Autodesk Fusion 360 part; units mm, degrees
(part 4 of 5)
  line L264 (61.2673, -37.956) -> (48.2686, -37.956)
  spline S265 degree 3 poles (48.2686, -37.956) (47.9937, -37.956) (47.7687, -37.7311) (47.7687, -37.456) knots 6 6 6 6 7 7 7 7
  line L265 (47.7687, -37.456) -> (47.7687, -24.4562)
  spline S266 degree 3 poles (4.9055, 32.6938) (4.9055, 32.9689) (5.1304, 33.1939) (5.4054, 33.1939) knots 0 0 0 0 1 1 1 1
  line L266 (5.4054, 33.1939) -> (18.4054, 33.1939)
  spline S267 degree 3 poles (18.4054, 33.1939) (18.6807, 33.1939) (18.9057, 32.9689) (18.9057, 32.6938) knots 2 2 2 2 3 3 3 3
  line L267 (18.9057, 32.6938) -> (18.9057, 19.6941)
  spline S268 degree 3 poles (18.9057, 19.6941) (18.9057, 19.419) (18.6807, 19.194) (18.4054, 19.194) knots 4 4 4 4 5 5 5 5
  line L268 (18.4054, 19.194) -> (5.4054, 19.194)
  spline S269 degree 3 poles (5.4054, 19.194) (5.1304, 19.194) (4.9055, 19.419) (4.9055, 19.6941) knots 6 6 6 6 7 7 7 7
  line L269 (4.9055, 19.6941) -> (4.9055, 32.6938)
  line L270 (-4.6195, 0.6441) -> (-4.6195, 13.6438)
  spline S270 degree 3 poles (-4.6195, 13.6438) (-4.6195, 13.9189) (-4.3946, 14.1438) (-4.1196, 14.1438) knots 1 1 1 1 2 2 2 2
  line L271 (-4.1196, 14.1438) -> (8.8804, 14.1438)
  spline S271 degree 3 poles (8.8804, 14.1438) (9.1557, 14.1438) (9.3807, 13.9189) (9.3807, 13.6438) knots 3 3 3 3 4 4 4 4
  line L272 (9.3807, 13.6438) -> (9.3807, 0.6441)
  spline S272 degree 3 poles (9.3807, 0.6441) (9.3807, 0.369) (9.1557, 0.144) (8.8804, 0.144) knots 5 5 5 5 6 6 6 6
  line L273 (8.8804, 0.144) -> (-4.1196, 0.144)
  spline S273 degree 3 poles (-4.1196, 0.144) (-4.3946, 0.144) (-4.6195, 0.369) (-4.6195, 0.6441) knots 7 7 7 7 8 8 8 8
  spline S274 degree 3 poles (-14.1445, 56.506) (-14.1445, 56.7811) (-13.9196, 57.006) (-13.6447, 57.006) knots 0 0 0 0 1 1 1 1
  line L274 (-13.6447, 57.006) -> (-0.6446, 57.006)
  spline S275 degree 3 poles (-0.6446, 57.006) (-0.3693, 57.006) (-0.1443, 56.7811) (-0.1443, 56.506) knots 2 2 2 2 3 3 3 3
  line L275 (-0.1443, 56.506) -> (-0.1443, 43.5059)
  spline S276 degree 3 poles (-0.1443, 43.5059) (-0.1443, 43.2308) (-0.3693, 43.0058) (-0.6446, 43.0058) knots 4 4 4 4 5 5 5 5
  line L276 (-0.6446, 43.0058) -> (-13.6447, 43.0058)
  spline S277 degree 3 poles (-13.6447, 43.0058) (-13.9196, 43.0058) (-14.1445, 43.2308) (-14.1445, 43.5059) knots 6 6 6 6 7 7 7 7
  line L277 (-14.1445, 43.5059) -> (-14.1445, 56.506)
  spline S278 degree 3 poles (-52.2446, 56.506) (-52.2446, 56.7811) (-52.0196, 57.006) (-51.7447, 57.006) knots 0 0 0 0 1 1 1 1
  line L278 (-51.7447, 57.006) -> (-38.7446, 57.006)
  spline S279 degree 3 poles (-38.7446, 57.006) (-38.4693, 57.006) (-38.2444, 56.7811) (-38.2444, 56.506) knots 2 2 2 2 3 3 3 3
  line L279 (-38.2444, 56.506) -> (-38.2444, 43.5059)
  spline S280 degree 3 poles (-38.2444, 43.5059) (-38.2444, 43.2308) (-38.4693, 43.0058) (-38.7446, 43.0058) knots 4 4 4 4 5 5 5 5
  line L280 (-38.7446, 43.0058) -> (-51.7447, 43.0058)
  spline S281 degree 3 poles (-51.7447, 43.0058) (-52.0196, 43.0058) (-52.2446, 43.2308) (-52.2446, 43.5059) knots 6 6 6 6 7 7 7 7
  line L281 (-52.2446, 43.5059) -> (-52.2446, 56.506)
  line L282 (-71.5816, 13.6438) -> (-71.5816, 0.6441)
  spline S282 degree 3 poles (-71.5816, 0.6441) (-71.5816, 0.369) (-71.8065, 0.144) (-72.0818, 0.144) knots 1 1 1 1 2 2 2 2
  line L283 (-72.0818, 0.144) -> (-85.0819, 0.144)
  spline S283 degree 3 poles (-85.0819, 0.144) (-85.3568, 0.144) (-85.5817, 0.369) (-85.5817, 0.6441) knots 3 3 3 3 4 4 4 4
  line L284 (-85.5817, 0.6441) -> (-85.5817, 13.6438)
  spline S284 degree 3 poles (-85.5817, 13.6438) (-85.5817, 13.9189) (-85.3568, 14.1438) (-85.0819, 14.1438) knots 5 5 5 5 6 6 6 6
  line L285 (-85.0819, 14.1438) -> (-72.0818, 14.1438)
  spline S285 degree 3 poles (-72.0818, 14.1438) (-71.8065, 14.1438) (-71.5816, 13.9189) (-71.5816, 13.6438) knots 7 7 7 7 8 8 8 8
  spline S286 degree 3 poles (-57.0067, -5.4062) (-57.0067, -5.1311) (-56.7818, -4.9062) (-56.5068, -4.9062) knots 0 0 0 0 1 1 1 1
  line L286 (-56.5068, -4.9062) -> (-43.5068, -4.9062)
  spline S287 degree 3 poles (-43.5068, -4.9062) (-43.2315, -4.9062) (-43.0065, -5.1311) (-43.0065, -5.4062) knots 2 2 2 2 3 3 3 3
  line L287 (-43.0065, -5.4062) -> (-43.0065, -18.406)
  spline S288 degree 3 poles (-43.0065, -18.406) (-43.0065, -18.681) (-43.2315, -18.906) (-43.5068, -18.906) knots 4 4 4 4 5 5 5 5
  line L288 (-43.5068, -18.906) -> (-56.5068, -18.906)
  spline S289 degree 3 poles (-56.5068, -18.906) (-56.7818, -18.906) (-57.0067, -18.681) (-57.0067, -18.406) knots 6 6 6 6 7 7 7 7
  line L289 (-57.0067, -18.406) -> (-57.0067, -5.4062)
  spline S290 degree 3 poles (43.0055, 56.506) (43.0055, 56.7811) (43.2305, 57.006) (43.5054, 57.006) knots 0 0 0 0 1 1 1 1
  line L290 (43.5054, 57.006) -> (56.5055, 57.006)
  spline S291 degree 3 poles (56.5055, 57.006) (56.7807, 57.006) (57.0057, 56.7811) (57.0057, 56.506) knots 2 2 2 2 3 3 3 3
  line L291 (57.0057, 56.506) -> (57.0057, 43.5059)
  spline S292 degree 3 poles (57.0057, 43.5059) (57.0057, 43.2308) (56.7807, 43.0058) (56.5055, 43.0058) knots 4 4 4 4 5 5 5 5
  line L292 (56.5055, 43.0058) -> (43.5054, 43.0058)
  spline S293 degree 3 poles (43.5054, 43.0058) (43.2305, 43.0058) (43.0055, 43.2308) (43.0055, 43.5059) knots 6 6 6 6 7 7 7 7
  line L293 (43.0055, 43.5059) -> (43.0055, 56.506)
  spline S294 degree 3 poles (38.7436, -18.906) (38.4687, -18.906) (38.2437, -18.681) (38.2437, -18.406) knots 0 0 0 0 1 1 1 1
  line L294 (38.2437, -18.406) -> (38.2437, -5.4062)
  spline S295 degree 3 poles (38.2437, -5.4062) (38.2437, -5.1311) (38.4687, -4.9062) (38.7436, -4.9062) knots 2 2 2 2 3 3 3 3
  line L295 (38.7436, -4.9062) -> (51.7433, -4.9062)
  spline S296 degree 3 poles (51.7433, -4.9062) (52.0186, -4.9062) (52.2435, -5.1311) (52.2435, -5.4062) knots 4 4 4 4 5 5 5 5
  line L296 (52.2435, -5.4062) -> (52.2435, -18.406)
  spline S297 degree 3 poles (52.2435, -18.406) (52.2435, -18.681) (52.0186, -18.906) (51.7433, -18.906) knots 6 6 6 6 7 7 7 7
  line L297 (51.7433, -18.906) -> (38.7436, -18.906)
  spline S298 degree 3 poles (-33.1946, 56.506) (-33.1946, 56.7811) (-32.9696, 57.006) (-32.6947, 57.006) knots 0 0 0 0 1 1 1 1
  line L298 (-32.6947, 57.006) -> (-19.6946, 57.006)
  spline S299 degree 3 poles (-19.6946, 57.006) (-19.4193, 57.006) (-19.1944, 56.7811) (-19.1944, 56.506) knots 2 2 2 2 3 3 3 3
  line L299 (-19.1944, 56.506) -> (-19.1944, 43.5059)
  spline S300 degree 3 poles (-19.1944, 43.5059) (-19.1944, 43.2308) (-19.4193, 43.0058) (-19.6946, 43.0058) knots 4 4 4 4 5 5 5 5
  line L300 (-19.6946, 43.0058) -> (-32.6947, 43.0058)
  spline S301 degree 3 poles (-32.6947, 43.0058) (-32.9696, 43.0058) (-33.1946, 43.2308) (-33.1946, 43.5059) knots 6 6 6 6 7 7 7 7
  line L301 (-33.1946, 43.5059) -> (-33.1946, 56.506)
  spline S302 degree 3 poles (-176.3566, -37.456) (-176.3566, -37.7311) (-176.5816, -37.956) (-176.8568, -37.956) knots 0 0 0 0 1 1 1 1
  line L302 (-176.8568, -37.956) -> (-189.8569, -37.956)
  spline S303 degree 3 poles (-189.8569, -37.956) (-190.1318, -37.956) (-190.3568, -37.7311) (-190.3568, -37.456) knots 2 2 2 2 3 3 3 3
  line L303 (-190.3568, -37.456) -> (-190.3568, -24.4562)
  spline S304 degree 3 poles (-190.3568, -24.4562) (-190.3568, -24.1811) (-190.1318, -23.9562) (-189.8569, -23.9562) knots 4 4 4 4 5 5 5 5
  line L304 (-189.8569, -23.9562) -> (-176.8568, -23.9562)
  spline S305 degree 3 poles (-176.8568, -23.9562) (-176.5816, -23.9562) (-176.3566, -24.1811) (-176.3566, -24.4562) knots 6 6 6 6 7 7 7 7
  line L305 (-176.3566, -24.4562) -> (-176.3566, -37.456)
  spline S306 degree 3 poles (-176.3566, 0.6441) (-176.3566, 0.369) (-176.5816, 0.144) (-176.8568, 0.144) knots 0 0 0 0 1 1 1 1
  line L306 (-176.8568, 0.144) -> (-189.8569, 0.144)
  spline S307 degree 3 poles (-189.8569, 0.144) (-190.1318, 0.144) (-190.3568, 0.369) (-190.3568, 0.6441) knots 2 2 2 2 3 3 3 3
  line L307 (-190.3568, 0.6441) -> (-190.3568, 13.6438)
  spline S308 degree 3 poles (-190.3568, 13.6438) (-190.3568, 13.9189) (-190.1318, 14.1438) (-189.8569, 14.1438) knots 4 4 4 4 5 5 5 5
  line L308 (-189.8569, 14.1438) -> (-176.8568, 14.1438)
  spline S309 degree 3 poles (-176.8568, 14.1438) (-176.5816, 14.1438) (-176.3566, 13.9189) (-176.3566, 13.6438) knots 6 6 6 6 7 7 7 7
  line L309 (-176.3566, 13.6438) -> (-176.3566, 0.6441)
  spline S310 degree 3 poles (57.7936, -18.906) (57.5187, -18.906) (57.2937, -18.681) (57.2937, -18.406) knots 0 0 0 0 1 1 1 1
  line L310 (57.2937, -18.406) -> (57.2937, -5.4062)
  spline S311 degree 3 poles (57.2937, -5.4062) (57.2937, -5.1311) (57.5187, -4.9062) (57.7936, -4.9062) knots 2 2 2 2 3 3 3 3
  line L311 (57.7936, -4.9062) -> (70.7933, -4.9062)
  spline S312 degree 3 poles (70.7933, -4.9062) (71.0686, -4.9062) (71.2935, -5.1311) (71.2935, -5.4062) knots 4 4 4 4 5 5 5 5
  line L312 (71.2935, -5.4062) -> (71.2935, -18.406)
  spline S313 degree 3 poles (71.2935, -18.406) (71.2935, -18.681) (71.0686, -18.906) (70.7933, -18.906) knots 6 6 6 6 7 7 7 7
  line L313 (70.7933, -18.906) -> (57.7936, -18.906)
  spline S314 degree 3 poles (95.3937, -5.4062) (95.3937, -5.1311) (95.6187, -4.9062) (95.8936, -4.9062) knots 0 0 0 0 1 1 1 1
  line L314 (95.8936, -4.9062) -> (108.8933, -4.9062)
  spline S315 degree 3 poles (108.8933, -4.9062) (109.1686, -4.9062) (109.3936, -5.1311) (109.3936, -5.4062) knots 2 2 2 2 3 3 3 3
  line L315 (109.3936, -5.4062) -> (109.3936, -18.406)
  spline S316 degree 3 poles (109.3936, -18.406) (109.3936, -18.681) (109.1686, -18.906) (108.8933, -18.906) knots 4 4 4 4 5 5 5 5
  line L316 (108.8933, -18.906) -> (95.8936, -18.906)
  spline S317 degree 3 poles (95.8936, -18.906) (95.6187, -18.906) (95.3937, -18.681) (95.3937, -18.406) knots 6 6 6 6 7 7 7 7
  line L317 (95.3937, -18.406) -> (95.3937, -5.4062)
  line L318 (33.4805, 0.6441) -> (33.4805, 13.6438)
  spline S318 degree 3 poles (33.4805, 13.6438) (33.4805, 13.9189) (33.7055, 14.1438) (33.9804, 14.1438) knots 1 1 1 1 2 2 2 2
  line L319 (33.9804, 14.1438) -> (46.9805, 14.1438)
  spline S319 degree 3 poles (46.9805, 14.1438) (47.2557, 14.1438) (47.4807, 13.9189) (47.4807, 13.6438) knots 3 3 3 3 4 4 4 4
  line L320 (47.4807, 13.6438) -> (47.4807, 0.6441)
  spline S320 degree 3 poles (47.4807, 0.6441) (47.4807, 0.369) (47.2557, 0.144) (46.9805, 0.144) knots 5 5 5 5 6 6 6 6
  line L321 (46.9805, 0.144) -> (33.9804, 0.144)
  spline S321 degree 3 poles (33.9804, 0.144) (33.7055, 0.144) (33.4805, 0.369) (33.4805, 0.6441) knots 7 7 7 7 8 8 8 8
  spline S322 degree 3 poles (-176.3566, 24.4559) (-176.3566, 24.1808) (-176.5816, 23.9558) (-176.8568, 23.9558) knots 0 0 0 0 1 1 1 1
  line L322 (-176.8568, 23.9558) -> (-189.8569, 23.9558)
  spline S323 degree 3 poles (-189.8569, 23.9558) (-190.1318, 23.9558) (-190.3568, 24.1808) (-190.3568, 24.4559) knots 2 2 2 2 3 3 3 3
  line L323 (-190.3568, 24.4559) -> (-190.3568, 37.456)
  spline S324 degree 3 poles (-190.3568, 37.456) (-190.3568, 37.7311) (-190.1318, 37.956) (-189.8569, 37.956) knots 4 4 4 4 5 5 5 5
  line L324 (-189.8569, 37.956) -> (-176.8568, 37.956)
  spline S325 degree 3 poles (-176.8568, 37.956) (-176.5816, 37.956) (-176.3566, 37.7311) (-176.3566, 37.456) knots 6 6 6 6 7 7 7 7
  line L325 (-176.3566, 37.456) -> (-176.3566, 24.4559)
  spline S326 degree 3 poles (28.7187, -24.4562) (28.7187, -24.1811) (28.9436, -23.9562) (29.2186, -23.9562) knots 0 0 0 0 1 1 1 1
  line L326 (29.2186, -23.9562) -> (42.2183, -23.9562)
  spline S327 degree 3 poles (42.2183, -23.9562) (42.4936, -23.9562) (42.7185, -24.1811) (42.7185, -24.4562) knots 2 2 2 2 3 3 3 3
  line L327 (42.7185, -24.4562) -> (42.7185, -37.456)
  spline S328 degree 3 poles (42.7185, -37.456) (42.7185, -37.7311) (42.4936, -37.956) (42.2183, -37.956) knots 4 4 4 4 5 5 5 5
  line L328 (42.2183, -37.956) -> (29.2186, -37.956)
  spline S329 degree 3 poles (29.2186, -37.956) (28.9436, -37.956) (28.7187, -37.7311) (28.7187, -37.456) knots 6 6 6 6 7 7 7 7
  line L329 (28.7187, -37.456) -> (28.7187, -24.4562)
  spline S330 degree 3 poles (43.0055, 32.6938) (43.0055, 32.9689) (43.2305, 33.1939) (43.5054, 33.1939) knots 0 0 0 0 1 1 1 1
  line L330 (43.5054, 33.1939) -> (56.5055, 33.1939)
  spline S331 degree 3 poles (56.5055, 33.1939) (56.7807, 33.1939) (57.0057, 32.9689) (57.0057, 32.6938) knots 2 2 2 2 3 3 3 3
  line L331 (57.0057, 32.6938) -> (57.0057, 19.6941)
  spline S332 degree 3 poles (57.0057, 19.6941) (57.0057, 19.419) (56.7807, 19.194) (56.5055, 19.194) knots 4 4 4 4 5 5 5 5
  line L332 (56.5055, 19.194) -> (43.5054, 19.194)
  spline S333 degree 3 poles (43.5054, 19.194) (43.2305, 19.194) (43.0055, 19.419) (43.0055, 19.6941) knots 6 6 6 6 7 7 7 7
  line L333 (43.0055, 19.6941) -> (43.0055, 32.6938)
  spline S334 degree 3 poles (-18.9064, -5.4062) (-18.9064, -5.1311) (-18.6814, -4.9062) (-18.4065, -4.9062) knots 0 0 0 0 1 1 1 1
  line L334 (-18.4065, -4.9062) -> (-5.4067, -4.9062)
  spline S335 degree 3 poles (-5.4067, -4.9062) (-5.1315, -4.9062) (-4.9065, -5.1311) (-4.9065, -5.4062) knots 2 2 2 2 3 3 3 3
  line L335 (-4.9065, -5.4062) -> (-4.9065, -18.406)
  spline S336 degree 3 poles (-4.9065, -18.406) (-4.9065, -18.681) (-5.1315, -18.906) (-5.4067, -18.906) knots 4 4 4 4 5 5 5 5
  line L336 (-5.4067, -18.906) -> (-18.4065, -18.906)
  spline S337 degree 3 poles (-18.4065, -18.906) (-18.6814, -18.906) (-18.9064, -18.681) (-18.9064, -18.406) knots 6 6 6 6 7 7 7 7
  line L337 (-18.9064, -18.406) -> (-18.9064, -5.4062)
  spline S338 degree 3 poles (-23.1697, 0.144) (-23.4446, 0.144) (-23.6695, 0.369) (-23.6695, 0.6441) knots 0 0 0 0 1 1 1 1
  line L338 (-23.6695, 0.6441) -> (-23.6695, 13.6438)
  spline S339 degree 3 poles (-23.6695, 13.6438) (-23.6695, 13.9189) (-23.4446, 14.1438) (-23.1697, 14.1438) knots 2 2 2 2 3 3 3 3
  line L339 (-23.1697, 14.1438) -> (-10.1696, 14.1438)
  spline S340 degree 3 poles (-10.1696, 14.1438) (-9.8943, 14.1438) (-9.6694, 13.9189) (-9.6694, 13.6438) knots 4 4 4 4 5 5 5 5
  line L340 (-9.6694, 13.6438) -> (-9.6694, 0.6441)
  spline S341 degree 3 poles (-9.6694, 0.6441) (-9.6694, 0.369) (-9.8943, 0.144) (-10.1696, 0.144) knots 6 6 6 6 7 7 7 7
  line L341 (-10.1696, 0.144) -> (-23.1697, 0.144)
  line L342 (-69.2006, -5.4062) -> (-69.2006, -18.406)
  spline S342 degree 3 poles (-69.2006, -18.406) (-69.2006, -18.681) (-69.4256, -18.906) (-69.7009, -18.906) knots 1 1 1 1 2 2 2 2
  line L343 (-69.7009, -18.906) -> (-82.7006, -18.906)
  spline S343 degree 3 poles (-82.7006, -18.906) (-82.9755, -18.906) (-83.2005, -18.681) (-83.2005, -18.406) knots 3 3 3 3 4 4 4 4
  line L344 (-83.2005, -18.406) -> (-83.2005, -5.4062)
  spline S344 degree 3 poles (-83.2005, -5.4062) (-83.2005, -5.1311) (-82.9755, -4.9062) (-82.7006, -4.9062) knots 5 5 5 5 6 6 6 6
  line L345 (-82.7006, -4.9062) -> (-69.7009, -4.9062)
  spline S345 degree 3 poles (-69.7009, -4.9062) (-69.4256, -4.9062) (-69.2006, -5.1311) (-69.2006, -5.4062) knots 7 7 7 7 8 8 8 8
  spline S346 degree 3 poles (-174.9321, 43.5059) (-174.9321, 43.2308) (-175.157, 43.0058) (-175.4323, 43.0058) knots 0 0 0 0 1 1 1 1
  line L346 (-175.4323, 43.0058) -> (-190.7823, 43.0058)
  spline S347 degree 3 poles (-190.7823, 43.0058) (-191.0572, 43.0058) (-191.2822, 43.2308) (-191.2822, 43.5059) knots 2 2 2 2 3 3 3 3
  line L347 (-191.2822, 43.5059) -> (-191.2822, 56.506)
  spline S348 degree 3 poles (-191.2822, 56.506) (-191.2822, 56.7811) (-191.0572, 57.006) (-190.7823, 57.006) knots 4 4 4 4 5 5 5 5
  line L348 (-190.7823, 57.006) -> (-175.4323, 57.006)
  spline S349 degree 3 poles (-175.4323, 57.006) (-175.157, 57.006) (-174.9321, 56.7811) (-174.9321, 56.506) knots 6 6 6 6 7 7 7 7
  line L349 (-174.9321, 56.506) -> (-174.9321, 43.5059)
  spline S350 degree 3 poles (-157.3066, -18.406) (-157.3066, -18.681) (-157.5316, -18.906) (-157.8068, -18.906) knots 0 0 0 0 1 1 1 1
  line L350 (-157.8068, -18.906) -> (-170.8069, -18.906)
  spline S351 degree 3 poles (-170.8069, -18.906) (-171.0818, -18.906) (-171.3068, -18.681) (-171.3068, -18.406) knots 2 2 2 2 3 3 3 3
  line L351 (-171.3068, -18.406) -> (-171.3068, -5.4062)
  spline S352 degree 3 poles (-171.3068, -5.4062) (-171.3068, -5.1311) (-171.0818, -4.9062) (-170.8069, -4.9062) knots 4 4 4 4 5 5 5 5
  line L352 (-170.8069, -4.9062) -> (-157.8068, -4.9062)
  spline S353 degree 3 poles (-157.8068, -4.9062) (-157.5316, -4.9062) (-157.3066, -5.1311) (-157.3066, -5.4062) knots 6 6 6 6 7 7 7 7
  line L353 (-157.3066, -5.4062) -> (-157.3066, -18.406)
  spline S354 degree 3 poles (-157.3066, -56.506) (-157.3066, -56.7811) (-157.5316, -57.006) (-157.8068, -57.006) knots 0 0 0 0 1 1 1 1
  line L354 (-157.8068, -57.006) -> (-170.8069, -57.006)
  spline S355 degree 3 poles (-170.8069, -57.006) (-171.0818, -57.006) (-171.3068, -56.7811) (-171.3068, -56.506) knots 2 2 2 2 3 3 3 3
  line L355 (-171.3068, -56.506) -> (-171.3068, -43.5062)
  spline S356 degree 3 poles (-171.3068, -43.5062) (-171.3068, -43.2312) (-171.0818, -43.0062) (-170.8069, -43.0062) knots 4 4 4 4 5 5 5 5
  line L356 (-170.8069, -43.0062) -> (-157.8068, -43.0062)
  spline S357 degree 3 poles (-157.8068, -43.0062) (-157.5316, -43.0062) (-157.3066, -43.2312) (-157.3066, -43.5062) knots 6 6 6 6 7 7 7 7
  line L357 (-157.3066, -43.5062) -> (-157.3066, -56.506)
  spline S358 degree 3 poles (-157.3066, 43.5059) (-157.3066, 43.2308) (-157.5316, 43.0058) (-157.8068, 43.0058) knots 0 0 0 0 1 1 1 1
  line L358 (-157.8068, 43.0058) -> (-170.8069, 43.0058)
  spline S359 degree 3 poles (-170.8069, 43.0058) (-171.0818, 43.0058) (-171.3068, 43.2308) (-171.3068, 43.5059) knots 2 2 2 2 3 3 3 3
  line L359 (-171.3068, 43.5059) -> (-171.3068, 56.506)
  spline S360 degree 3 poles (-171.3068, 56.506) (-171.3068, 56.7811) (-171.0818, 57.006) (-170.8069, 57.006) knots 4 4 4 4 5 5 5 5
  line L360 (-170.8069, 57.006) -> (-157.8068, 57.006)
  spline S361 degree 3 poles (-157.8068, 57.006) (-157.5316, 57.006) (-157.3066, 56.7811) (-157.3066, 56.506) knots 6 6 6 6 7 7 7 7
  line L361 (-157.3066, 56.506) -> (-157.3066, 43.5059)
  spline S362 degree 3 poles (-14.1445, 32.6938) (-14.1445, 32.9689) (-13.9196, 33.1939) (-13.6447, 33.1939) knots 0 0 0 0 1 1 1 1
  line L362 (-13.6447, 33.1939) -> (-0.6446, 33.1939)
  spline S363 degree 3 poles (-0.6446, 33.1939) (-0.3693, 33.1939) (-0.1443, 32.9689) (-0.1443, 32.6938) knots 2 2 2 2 3 3 3 3
  line L363 (-0.1443, 32.6938) -> (-0.1443, 19.6941)
  spline S364 degree 3 poles (-0.1443, 19.6941) (-0.1443, 19.419) (-0.3693, 19.194) (-0.6446, 19.194) knots 4 4 4 4 5 5 5 5
  line L364 (-0.6446, 19.194) -> (-13.6447, 19.194)
  spline S365 degree 3 poles (-13.6447, 19.194) (-13.9196, 19.194) (-14.1445, 19.419) (-14.1445, 19.6941) knots 6 6 6 6 7 7 7 7
  line L365 (-14.1445, 19.6941) -> (-14.1445, 32.6938)
  spline S366 degree 3 poles (-138.2566, -18.406) (-138.2566, -18.681) (-138.4816, -18.906) (-138.7568, -18.906) knots 0 0 0 0 1 1 1 1
  line L366 (-138.7568, -18.906) -> (-151.7569, -18.906)
  spline S367 degree 3 poles (-151.7569, -18.906) (-152.0318, -18.906) (-152.2568, -18.681) (-152.2568, -18.406) knots 2 2 2 2 3 3 3 3
  line L367 (-152.2568, -18.406) -> (-152.2568, -5.4062)
  spline S368 degree 3 poles (-152.2568, -5.4062) (-152.2568, -5.1311) (-152.0318, -4.9062) (-151.7569, -4.9062) knots 4 4 4 4 5 5 5 5
  line L368 (-151.7569, -4.9062) -> (-138.7568, -4.9062)
  spline S369 degree 3 poles (-138.7568, -4.9062) (-138.4816, -4.9062) (-138.2566, -5.1311) (-138.2566, -5.4062) knots 6 6 6 6 7 7 7 7
  line L369 (-138.2566, -5.4062) -> (-138.2566, -18.406)
  spline S370 degree 3 poles (-100.1566, -18.406) (-100.1566, -18.681) (-100.3815, -18.906) (-100.6568, -18.906) knots 0 0 0 0 1 1 1 1
  line L370 (-100.6568, -18.906) -> (-113.6569, -18.906)
  spline S371 degree 3 poles (-113.6569, -18.906) (-113.9318, -18.906) (-114.1568, -18.681) (-114.1568, -18.406) knots 2 2 2 2 3 3 3 3
  line L371 (-114.1568, -18.406) -> (-114.1568, -5.4062)
  spline S372 degree 3 poles (-114.1568, -5.4062) (-114.1568, -5.1311) (-113.9318, -4.9062) (-113.6569, -4.9062) knots 4 4 4 4 5 5 5 5
  line L372 (-113.6569, -4.9062) -> (-100.6568, -4.9062)
  spline S373 degree 3 poles (-100.6568, -4.9062) (-100.3815, -4.9062) (-100.1566, -5.1311) (-100.1566, -5.4062) knots 6 6 6 6 7 7 7 7
  line L373 (-100.1566, -5.4062) -> (-100.1566, -18.406)
  spline S374 degree 3 poles (-33.4815, -37.456) (-33.4815, -37.7311) (-33.7065, -37.956) (-33.9818, -37.956) knots 0 0 0 0 1 1 1 1
  line L374 (-33.9818, -37.956) -> (-46.9815, -37.956)
  spline S375 degree 3 poles (-46.9815, -37.956) (-47.2564, -37.956) (-47.4814, -37.7311) (-47.4814, -37.456) knots 2 2 2 2 3 3 3 3
  line L375 (-47.4814, -37.456) -> (-47.4814, -24.4562)
  spline S376 degree 3 poles (-47.4814, -24.4562) (-47.4814, -24.1811) (-47.2564, -23.9562) (-46.9815, -23.9562) knots 4 4 4 4 5 5 5 5
  line L376 (-46.9815, -23.9562) -> (-33.9818, -23.9562)
  spline S377 degree 3 poles (-33.9818, -23.9562) (-33.7065, -23.9562) (-33.4815, -24.1811) (-33.4815, -24.4562) knots 6 6 6 6 7 7 7 7
  line L377 (-33.4815, -24.4562) -> (-33.4815, -37.456)
  spline S378 degree 3 poles (-100.1566, 24.4559) (-100.1566, 24.1808) (-100.3815, 23.9558) (-100.6568, 23.9558) knots 0 0 0 0 1 1 1 1
  line L378 (-100.6568, 23.9558) -> (-113.6569, 23.9558)
  spline S379 degree 3 poles (-113.6569, 23.9558) (-113.9318, 23.9558) (-114.1568, 24.1808) (-114.1568, 24.4559) knots 2 2 2 2 3 3 3 3
  line L379 (-114.1568, 24.4559) -> (-114.1568, 37.456)
  spline S380 degree 3 poles (-114.1568, 37.456) (-114.1568, 37.7311) (-113.9318, 37.956) (-113.6569, 37.956) knots 4 4 4 4 5 5 5 5
  line L380 (-113.6569, 37.956) -> (-100.6568, 37.956)
  spline S381 degree 3 poles (-100.6568, 37.956) (-100.3815, 37.956) (-100.1566, 37.7311) (-100.1566, 37.456) knots 6 6 6 6 7 7 7 7
  line L381 (-100.1566, 37.456) -> (-100.1566, 24.4559)
  spline S382 degree 3 poles (-38.2444, -56.506) (-38.2444, -56.7811) (-38.4693, -57.006) (-38.7446, -57.006) knots 0 0 0 0 1 1 1 1
  line L382 (-38.7446, -57.006) -> (-51.7447, -57.006)
  spline S383 degree 3 poles (-51.7447, -57.006) (-52.0196, -57.006) (-52.2446, -56.7811) (-52.2446, -56.506) knots 2 2 2 2 3 3 3 3
  line L383 (-52.2446, -56.506) -> (-52.2446, -43.5062)
  spline S384 degree 3 poles (-52.2446, -43.5062) (-52.2446, -43.2312) (-52.0196, -43.0062) (-51.7447, -43.0062) knots 4 4 4 4 5 5 5 5
  line L384 (-51.7447, -43.0062) -> (-38.7446, -43.0062)
  spline S385 degree 3 poles (-38.7446, -43.0062) (-38.4693, -43.0062) (-38.2444, -43.2312) (-38.2444, -43.5062) knots 6 6 6 6 7 7 7 7
  line L385 (-38.2444, -43.5062) -> (-38.2444, -56.506)
  spline S386 degree 3 poles (-57.2947, -56.506) (-57.2947, -56.7811) (-57.5197, -57.006) (-57.795, -57.006) knots 0 0 0 0 1 1 1 1
  line L386 (-57.795, -57.006) -> (-70.7947, -57.006)
  spline S387 degree 3 poles (-70.7947, -57.006) (-71.0696, -57.006) (-71.2946, -56.7811) (-71.2946, -56.506) knots 2 2 2 2 3 3 3 3
  line L387 (-71.2946, -56.506) -> (-71.2946, -43.5062)
  spline S388 degree 3 poles (-71.2946, -43.5062) (-71.2946, -43.2312) (-71.0696, -43.0062) (-70.7947, -43.0062) knots 4 4 4 4 5 5 5 5
  line L388 (-70.7947, -43.0062) -> (-57.795, -43.0062)
  spline S389 degree 3 poles (-57.795, -43.0062) (-57.5197, -43.0062) (-57.2947, -43.2312) (-57.2947, -43.5062) knots 6 6 6 6 7 7 7 7
  line L389 (-57.2947, -43.5062) -> (-57.2947, -56.506)
  spline S390 degree 3 poles (152.2558, -56.506) (152.2558, -56.7811) (152.0308, -57.006) (151.7555, -57.006) knots 0 0 0 0 1 1 1 1
  line L390 (151.7555, -57.006) -> (138.7554, -57.006)
  spline S391 degree 3 poles (138.7554, -57.006) (138.4805, -57.006) (138.2556, -56.7811) (138.2556, -56.506) knots 2 2 2 2 3 3 3 3
  line L391 (138.2556, -56.506) -> (138.2556, -43.5062)
  spline S392 degree 3 poles (138.2556, -43.5062) (138.2556, -43.2312) (138.4805, -43.0062) (138.7554, -43.0062) knots 4 4 4 4 5 5 5 5
  line L392 (138.7554, -43.0062) -> (151.7555, -43.0062)
  spline S393 degree 3 poles (151.7555, -43.0062) (152.0308, -43.0062) (152.2558, -43.2312) (152.2558, -43.5062) knots 6 6 6 6 7 7 7 7
  line L393 (152.2558, -43.5062) -> (152.2558, -56.506)
  spline S394 degree 3 poles (-19.1944, -56.506) (-19.1944, -56.7811) (-19.4193, -57.006) (-19.6946, -57.006) knots 0 0 0 0 1 1 1 1
  line L394 (-19.6946, -57.006) -> (-32.6947, -57.006)
  spline S395 degree 3 poles (-32.6947, -57.006) (-32.9696, -57.006) (-33.1946, -56.7811) (-33.1946, -56.506) knots 2 2 2 2 3 3 3 3
  line L395 (-33.1946, -56.506) -> (-33.1946, -43.5062)
  spline S396 degree 3 poles (-33.1946, -43.5062) (-33.1946, -43.2312) (-32.9696, -43.0062) (-32.6947, -43.0062) knots 4 4 4 4 5 5 5 5
  line L396 (-32.6947, -43.0062) -> (-19.6946, -43.0062)
  spline S397 degree 3 poles (-19.6946, -43.0062) (-19.4193, -43.0062) (-19.1944, -43.2312) (-19.1944, -43.5062) knots 6 6 6 6 7 7 7 7
  line L397 (-19.1944, -43.5062) -> (-19.1944, -56.506)
  spline S398 degree 3 poles (114.1557, -56.506) (114.1557, -56.7811) (113.9308, -57.006) (113.6555, -57.006) knots 0 0 0 0 1 1 1 1
  line L398 (113.6555, -57.006) -> (100.6554, -57.006)
  spline S399 degree 3 poles (100.6554, -57.006) (100.3805, -57.006) (100.1555, -56.7811) (100.1555, -56.506) knots 2 2 2 2 3 3 3 3
  line L399 (100.1555, -56.506) -> (100.1555, -43.5062)
  spline S400 degree 3 poles (100.1555, -43.5062) (100.1555, -43.2312) (100.3805, -43.0062) (100.6554, -43.0062) knots 4 4 4 4 5 5 5 5
  line L400 (100.6554, -43.0062) -> (113.6555, -43.0062)
  spline S401 degree 3 poles (113.6555, -43.0062) (113.9308, -43.0062) (114.1557, -43.2312) (114.1557, -43.5062) knots 6 6 6 6 7 7 7 7
  line L401 (114.1557, -43.5062) -> (114.1557, -56.506)
  spline S402 degree 3 poles (171.3058, -56.506) (171.3058, -56.7811) (171.0808, -57.006) (170.8055, -57.006) knots 0 0 0 0 1 1 1 1
  line L402 (170.8055, -57.006) -> (157.8055, -57.006)
  spline S403 degree 3 poles (157.8055, -57.006) (157.5305, -57.006) (157.3056, -56.7811) (157.3056, -56.506) knots 2 2 2 2 3 3 3 3
  line L403 (157.3056, -56.506) -> (157.3056, -43.5062)
  spline S404 degree 3 poles (157.3056, -43.5062) (157.3056, -43.2312) (157.5305, -43.0062) (157.8055, -43.0062) knots 4 4 4 4 5 5 5 5
  line L404 (157.8055, -43.0062) -> (170.8055, -43.0062)
  spline S405 degree 3 poles (170.8055, -43.0062) (171.0808, -43.0062) (171.3058, -43.2312) (171.3058, -43.5062) knots 6 6 6 6 7 7 7 7
  line L405 (171.3058, -43.5062) -> (171.3058, -56.506)
  spline S406 degree 3 poles (-100.1566, -37.456) (-100.1566, -37.7311) (-100.3815, -37.956) (-100.6568, -37.956) knots 0 0 0 0 1 1 1 1
  line L406 (-100.6568, -37.956) -> (-113.6569, -37.956)
  spline S407 degree 3 poles (-113.6569, -37.956) (-113.9318, -37.956) (-114.1568, -37.7311) (-114.1568, -37.456) knots 2 2 2 2 3 3 3 3
  line L407 (-114.1568, -37.456) -> (-114.1568, -24.4562)
  spline S408 degree 3 poles (-114.1568, -24.4562) (-114.1568, -24.1811) (-113.9318, -23.9562) (-113.6569, -23.9562) knots 4 4 4 4 5 5 5 5
  line L408 (-113.6569, -23.9562) -> (-100.6568, -23.9562)
  spline S409 degree 3 poles (-100.6568, -23.9562) (-100.3815, -23.9562) (-100.1566, -24.1811) (-100.1566, -24.4562) knots 6 6 6 6 7 7 7 7
  line L409 (-100.1566, -24.4562) -> (-100.1566, -37.456)
  spline S410 degree 3 poles (-119.2066, 0.6441) (-119.2066, 0.369) (-119.4315, 0.144) (-119.7068, 0.144) knots 0 0 0 0 1 1 1 1
  line L410 (-119.7068, 0.144) -> (-132.7069, 0.144)
  spline S411 degree 3 poles (-132.7069, 0.144) (-132.9818, 0.144) (-133.2068, 0.369) (-133.2068, 0.6441) knots 2 2 2 2 3 3 3 3
  line L411 (-133.2068, 0.6441) -> (-133.2068, 13.6438)
  spline S412 degree 3 poles (-133.2068, 13.6438) (-133.2068, 13.9189) (-132.9818, 14.1438) (-132.7069, 14.1438) knots 4 4 4 4 5 5 5 5
  line L412 (-132.7069, 14.1438) -> (-119.7068, 14.1438)
  spline S413 degree 3 poles (-119.7068, 14.1438) (-119.4315, 14.1438) (-119.2066, 13.9189) (-119.2066, 13.6438) knots 6 6 6 6 7 7 7 7
  line L413 (-119.2066, 13.6438) -> (-119.2066, 0.6441)
  spline S414 degree 3 poles (99.8686, -37.456) (99.8686, -37.7311) (99.6436, -37.956) (99.3683, -37.956) knots 0 0 0 0 1 1 1 1
  line L414 (99.3683, -37.956) -> (86.3686, -37.956)
  spline S415 degree 3 poles (86.3686, -37.956) (86.0937, -37.956) (85.8687, -37.7311) (85.8687, -37.456) knots 2 2 2 2 3 3 3 3
  line L415 (85.8687, -37.456) -> (85.8687, -24.4562)
  spline S416 degree 3 poles (85.8687, -24.4562) (85.8687, -24.1811) (86.0937, -23.9562) (86.3686, -23.9562) knots 4 4 4 4 5 5 5 5
  line L416 (86.3686, -23.9562) -> (99.3683, -23.9562)
  spline S417 degree 3 poles (99.3683, -23.9562) (99.6436, -23.9562) (99.8686, -24.1811) (99.8686, -24.4562) knots 6 6 6 6 7 7 7 7
  line L417 (99.8686, -24.4562) -> (99.8686, -37.456)
  spline S418 degree 3 poles (92.1805, -51.8062) (92.1805, -52.0813) (92.0509, -52.3062) (91.7347, -52.3062) (91.6051, -52.5312) (91.6051, -52.8063) knots 0 0 0 0 1 1 2 2 2 2
  line L418 (91.6051, -52.8063) -> (91.6051, -55.536)
  spline S419 degree 3 poles (91.6051, -55.536) (91.6051, -55.8111) (91.3802, -56.0361) (91.1049, -56.0361) knots 3 3 3 3 4 4 4 4
  line L419 (91.1049, -56.0361) -> (85.005, -56.0361)
  spline S420 degree 3 poles (85.005, -56.0361) (84.7301, -56.0361) (84.5051, -55.8111) (84.5051, -55.536) knots 5 5 5 5 6 6 6 6
  line L420 (84.5051, -55.536) -> (84.5051, -52.8063)
  spline S421 degree 3 poles (84.5051, -52.8063) (84.5051, -52.5312) (84.2802, -52.3062) (84.0049, -52.3062) knots 7 7 7 7 8 8 8 8
  line L421 (84.0049, -52.3062) -> (47.9802, -52.3062)
  spline S422 degree 3 poles (47.9802, -52.3062) (47.7053, -52.3062) (47.4803, -52.5312) (47.4803, -52.8063) knots 9 9 9 9 10 10 10 10
  line L422 (47.4803, -52.8063) -> (47.4803, -56.506)
  spline S423 degree 3 poles (47.4803, -56.506) (47.4803, -56.7811) (47.2554, -57.006) (46.9801, -57.006) knots 11 11 11 11 12 12 12 12
  line L423 (46.9801, -57.006) -> (33.98, -57.006)
  spline S424 degree 3 poles (33.98, -57.006) (33.7051, -57.006) (33.4801, -56.7811) (33.4801, -56.506) knots 13 13 13 13 14 14 14 14
  line L424 (33.4801, -56.506) -> (33.4801, -52.8063)
  spline S425 degree 3 poles (33.4801, -52.8063) (33.4801, -52.5312) (33.2552, -52.3062) (32.9799, -52.3062) knots 15 15 15 15 16 16 16 16
  line L425 (32.9799, -52.3062) -> (-3.0451, -52.3062)
  spline S426 degree 3 poles (-3.0451, -52.3062) (-3.32, -52.3062) (-3.545, -52.5312) (-3.545, -52.8063) knots 17 17 17 17 18 18 18 18
  line L426 (-3.545, -52.8063) -> (-3.545, -55.536)
  spline S427 degree 3 poles (-3.545, -55.536) (-3.545, -55.8111) (-3.77, -56.0361) (-4.0452, -56.0361) knots 19 19 19 19 20 20 20 20
  line L427 (-4.0452, -56.0361) -> (-10.1451, -56.0361)
  spline S428 degree 3 poles (-10.1451, -56.0361) (-10.42, -56.0361) (-10.645, -55.8111) (-10.645, -55.536) knots 21 21 21 21 22 22 22 22
  line L428 (-10.645, -55.536) -> (-10.645, -52.8063)
  spline S429 degree 3 poles (-10.645, -52.8063) (-10.645, -52.5312) (-10.7745, -52.3062) (-10.9323, -52.3062) (-11.0905, -52.3062) (-11.2196, -52.0813) (-11.2196, -51.8062) knots 23 23 23 23 24 24 24 25 25 25 25
  line L429 (-11.2196, -51.8062) -> (-11.2196, -50.0061)
  spline S430 degree 3 poles (-11.2196, -50.0061) (-11.2196, -49.731) (-11.0905, -49.5061) (-10.9323, -49.5061) (-10.7745, -49.5061) (-10.645, -49.2811) (-10.645, -49.006) knots 26 26 26 26 27 27 27 28 28 28 28
  line L430 (-10.645, -49.006) -> (-10.645, -43.7364)
  spline S431 degree 3 poles (-10.645, -43.7364) (-10.645, -43.4613) (-10.42, -43.2363) (-10.1451, -43.2363) knots 29 29 29 29 30 30 30 30
  line L431 (-10.1451, -43.2363) -> (-9.4203, -43.2363)
  spline S432 degree 3 poles (-9.4203, -43.2363) (-9.145, -43.2363) (-8.92, -43.0114) (-8.92, -42.7363) knots 31 31 31 31 32 32 32 32
  line L432 (-8.92, -42.7363) -> (-8.92, -42.5361)
  spline S433 degree 3 poles (-8.92, -42.5361) (-8.92, -42.261) (-8.6951, -42.036) (-8.4202, -42.036) knots 33 33 33 33 34 34 34 34
  line L433 (-8.4202, -42.036) -> (-5.7702, -42.036)
  spline S434 degree 3 poles (-5.7702, -42.036) (-5.4949, -42.036) (-5.27, -42.261) (-5.27, -42.5361) knots 35 35 35 35 36 36 36 36
  line L434 (-5.27, -42.5361) -> (-5.27, -42.7363)
  spline S435 degree 3 poles (-5.27, -42.7363) (-5.27, -43.0114) (-5.045, -43.2363) (-4.7701, -43.2363) knots 37 37 37 37 38 38 38 38
  line L435 (-4.7701, -43.2363) -> (-4.0452, -43.2363)
  spline S436 degree 3 poles (-4.0452, -43.2363) (-3.77, -43.2363) (-3.545, -43.4613) (-3.545, -43.7364) knots 39 39 39 39 40 40 40 40
  line L436 (-3.545, -43.7364) -> (-3.545, -47.2063)
  spline S437 degree 3 poles (-3.545, -47.2063) (-3.545, -47.4814) (-3.32, -47.7063) (-3.0451, -47.7063) knots 41 41 41 41 42 42 42 42
  line L437 (-3.0451, -47.7063) -> (32.9799, -47.7063)
  spline S438 degree 3 poles (32.9799, -47.7063) (33.2552, -47.7063) (33.4801, -47.4814) (33.4801, -47.2063) knots 43 43 43 43 44 44 44 44
  line L438 (33.4801, -47.2063) -> (33.4801, -43.5062)
  spline S439 degree 3 poles (33.4801, -43.5062) (33.4801, -43.2312) (33.7051, -43.0062) (33.98, -43.0062) knots 45 45 45 45 46 46 46 46
  line L439 (33.98, -43.0062) -> (46.9801, -43.0062)
  spline S440 degree 3 poles (46.9801, -43.0062) (47.2554, -43.0062) (47.4803, -43.2312) (47.4803, -43.5062) knots 47 47 47 47 48 48 48 48
  line L440 (47.4803, -43.5062) -> (47.4803, -47.2063)
  spline S441 degree 3 poles (47.4803, -47.2063) (47.4803, -47.4814) (47.7053, -47.7063) (47.9802, -47.7063) knots 49 49 49 49 50 50 50 50
  line L441 (47.9802, -47.7063) -> (84.0049, -47.7063)
  spline S442 degree 3 poles (84.0049, -47.7063) (84.2802, -47.7063) (84.5051, -47.4814) (84.5051, -47.2063) knots 51 51 51 51 52 52 52 52
  line L442 (84.5051, -47.2063) -> (84.5051, -43.7364)
  spline S443 degree 3 poles (84.5051, -43.7364) (84.5051, -43.4613) (84.7301, -43.2363) (85.005, -43.2363) knots 53 53 53 53 54 54 54 54
  line L443 (85.005, -43.2363) -> (85.7299, -43.2363)
  spline S444 degree 3 poles (85.7299, -43.2363) (86.0051, -43.2363) (86.2301, -43.0114) (86.2301, -42.7363) knots 55 55 55 55 56 56 56 56
  line L444 (86.2301, -42.7363) -> (86.2301, -42.5361)
  spline S445 degree 3 poles (86.2301, -42.5361) (86.2301, -42.261) (86.4551, -42.036) (86.73, -42.036) knots 57 57 57 57 58 58 58 58
  line L445 (86.73, -42.036) -> (89.38, -42.036)
  spline S446 degree 3 poles (89.38, -42.036) (89.6549, -42.036) (89.8798, -42.261) (89.8798, -42.5361) knots 59 59 59 59 60 60 60 60
  line L446 (89.8798, -42.5361) -> (89.8798, -42.7363)
  spline S447 degree 3 poles (89.8798, -42.7363) (89.8798, -43.0114) (90.1048, -43.2363) (90.3801, -43.2363) knots 61 61 61 61 62 62 62 62
  line L447 (90.3801, -43.2363) -> (91.1049, -43.2363)
  spline S448 degree 3 poles (91.1049, -43.2363) (91.3802, -43.2363) (91.6051, -43.4613) (91.6051, -43.7364) knots 63 63 63 63 64 64 64 64
  line L448 (91.6051, -43.7364) -> (91.6051, -49.006)
  spline S449 degree 3 poles (91.6051, -49.006) (91.6051, -49.2811) (91.7347, -49.5061) (92.0509, -49.5061) (92.1805, -49.731) (92.1805, -50.0061) knots 65 65 65 65 66 66 67 67 67 67
  line L449 (92.1805, -50.0061) -> (92.1805, -51.8062)
  spline S450 degree 3 poles (133.2057, -56.506) (133.2057, -56.7811) (132.9808, -57.006) (132.7055, -57.006) knots 0 0 0 0 1 1 1 1
  line L450 (132.7055, -57.006) -> (119.7054, -57.006)
  spline S451 degree 3 poles (119.7054, -57.006) (119.4305, -57.006) (119.2056, -56.7811) (119.2056, -56.506) knots 2 2 2 2 3 3 3 3
  line L451 (119.2056, -56.506) -> (119.2056, -43.5062)
  spline S452 degree 3 poles (119.2056, -43.5062) (119.2056, -43.2312) (119.4305, -43.0062) (119.7054, -43.0062) knots 4 4 4 4 5 5 5 5
  line L452 (119.7054, -43.0062) -> (132.7055, -43.0062)
  spline S453 degree 3 poles (132.7055, -43.0062) (132.9808, -43.0062) (133.2057, -43.2312) (133.2057, -43.5062) knots 6 6 6 6 7 7 7 7
  line L453 (133.2057, -43.5062) -> (133.2057, -56.506)
  spline S454 degree 3 poles (-119.2066, -18.406) (-119.2066, -18.681) (-119.4315, -18.906) (-119.7068, -18.906) knots 0 0 0 0 1 1 1 1
  line L454 (-119.7068, -18.906) -> (-132.7069, -18.906)
  spline S455 degree 3 poles (-132.7069, -18.906) (-132.9818, -18.906) (-133.2068, -18.681) (-133.2068, -18.406) knots 2 2 2 2 3 3 3 3
  line L455 (-133.2068, -18.406) -> (-133.2068, -5.4062)
  spline S456 degree 3 poles (-133.2068, -5.4062) (-133.2068, -5.1311) (-132.9818, -4.9062) (-132.7069, -4.9062) knots 4 4 4 4 5 5 5 5
  line L456 (-132.7069, -4.9062) -> (-119.7068, -4.9062)
  spline S457 degree 3 poles (-119.7068, -4.9062) (-119.4315, -4.9062) (-119.2066, -5.1311) (-119.2066, -5.4062) knots 6 6 6 6 7 7 7 7
  line L457 (-119.2066, -5.4062) -> (-119.2066, -18.406)
  spline S458 degree 3 poles (-14.4315, -37.456) (-14.4315, -37.7311) (-14.6565, -37.956) (-14.9317, -37.956) knots 0 0 0 0 1 1 1 1
  line L458 (-14.9317, -37.956) -> (-27.9315, -37.956)
  spline S459 degree 3 poles (-27.9315, -37.956) (-28.2064, -37.956) (-28.4314, -37.7311) (-28.4314, -37.456) knots 2 2 2 2 3 3 3 3
  line L459 (-28.4314, -37.456) -> (-28.4314, -24.4562)
  spline S460 degree 3 poles (-28.4314, -24.4562) (-28.4314, -24.1811) (-28.2064, -23.9562) (-27.9315, -23.9562) knots 4 4 4 4 5 5 5 5
  line L460 (-27.9315, -23.9562) -> (-14.9317, -23.9562)
  spline S461 degree 3 poles (-14.9317, -23.9562) (-14.6565, -23.9562) (-14.4315, -24.1811) (-14.4315, -24.4562) knots 6 6 6 6 7 7 7 7
  line L461 (-14.4315, -24.4562) -> (-14.4315, -37.456)
  spline S462 degree 3 poles (-100.1566, 43.5059) (-100.1566, 43.2308) (-100.3815, 43.0058) (-100.6568, 43.0058) knots 0 0 0 0 1 1 1 1
  line L462 (-100.6568, 43.0058) -> (-113.6569, 43.0058)
  spline S463 degree 3 poles (-113.6569, 43.0058) (-113.9318, 43.0058) (-114.1568, 43.2308) (-114.1568, 43.5059) knots 2 2 2 2 3 3 3 3
  line L463 (-114.1568, 43.5059) -> (-114.1568, 56.506)
  spline S464 degree 3 poles (-114.1568, 56.506) (-114.1568, 56.7811) (-113.9318, 57.006) (-113.6569, 57.006) knots 4 4 4 4 5 5 5 5
  line L464 (-113.6569, 57.006) -> (-100.6568, 57.006)
  spline S465 degree 3 poles (-100.6568, 57.006) (-100.3815, 57.006) (-100.1566, 56.7811) (-100.1566, 56.506) knots 6 6 6 6 7 7 7 7
  line L465 (-100.1566, 56.506) -> (-100.1566, 43.5059)
  spline S466 degree 3 poles (-76.3447, -56.506) (-76.3447, -56.7811) (-76.5697, -57.006) (-76.845, -57.006) knots 0 0 0 0 1 1 1 1
  line L466 (-76.845, -57.006) -> (-89.8447, -57.006)
  spline S467 degree 3 poles (-89.8447, -57.006) (-90.1196, -57.006) (-90.3446, -56.7811) (-90.3446, -56.506) knots 2 2 2 2 3 3 3 3
  line L467 (-90.3446, -56.506) -> (-90.3446, -43.5062)
  spline S468 degree 3 poles (-90.3446, -43.5062) (-90.3446, -43.2312) (-90.1196, -43.0062) (-89.8447, -43.0062) knots 4 4 4 4 5 5 5 5
  line L468 (-89.8447, -43.0062) -> (-76.845, -43.0062)
  spline S469 degree 3 poles (-76.845, -43.0062) (-76.5697, -43.0062) (-76.3447, -43.2312) (-76.3447, -43.5062) knots 6 6 6 6 7 7 7 7
  line L469 (-76.3447, -43.5062) -> (-76.3447, -56.506)
  spline S470 degree 3 poles (118.9186, -37.456) (118.9186, -37.7311) (118.6936, -37.956) (118.4183, -37.956) knots 0 0 0 0 1 1 1 1
  line L470 (118.4183, -37.956) -> (105.4186, -37.956)
  spline S471 degree 3 poles (105.4186, -37.956) (105.1437, -37.956) (104.9187, -37.7311) (104.9187, -37.456) knots 2 2 2 2 3 3 3 3
  line L471 (104.9187, -37.456) -> (104.9187, -24.4562)
  spline S472 degree 3 poles (104.9187, -24.4562) (104.9187, -24.1811) (105.1437, -23.9562) (105.4186, -23.9562) knots 4 4 4 4 5 5 5 5
  line L472 (105.4186, -23.9562) -> (118.4183, -23.9562)
  spline S473 degree 3 poles (118.4183, -23.9562) (118.6936, -23.9562) (118.9186, -24.1811) (118.9186, -24.4562) knots 6 6 6 6 7 7 7 7
  line L473 (118.9186, -24.4562) -> (118.9186, -37.456)
  spline S474 degree 3 poles (-52.5315, -37.456) (-52.5315, -37.7311) (-52.7565, -37.956) (-53.0318, -37.956) knots 0 0 0 0 1 1 1 1
  line L474 (-53.0318, -37.956) -> (-57.139, -37.956)
  spline S475 degree 3 poles (-57.139, -37.956) (-57.4143, -37.956) (-57.6392, -38.1743) (-57.6392, -38.7079) (-57.8642, -38.9262) (-58.1391, -38.9262) knots 2 2 2 2 3 3 4 4 4 4
  line L475 (-58.1391, -38.9262) -> (-60.7891, -38.9262)
  spline S476 degree 3 poles (-60.7891, -38.9262) (-61.064, -38.9262) (-61.289, -38.7079) (-61.289, -38.1743) (-61.5139, -37.956) (-61.7892, -37.956) knots 5 5 5 5 6 6 7 7 7 7
  line L476 (-61.7892, -37.956) -> (-81.089, -37.956)
  spline S477 degree 3 poles (-81.089, -37.956) (-81.3643, -37.956) (-81.5892, -38.1743) (-81.5892, -38.7079) (-81.8142, -38.9262) (-82.0891, -38.9262) knots 8 8 8 8 9 9 10 10 10 10
  line L477 (-82.0891, -38.9262) -> (-84.738, -38.9262)
  spline S478 degree 3 poles (-84.738, -38.9262) (-85.0133, -38.9262) (-85.2383, -38.7079) (-85.2383, -38.1743) (-85.4632, -37.956) (-85.7381, -37.956) knots 11 11 11 11 12 12 13 13 13 13
  line L478 (-85.7381, -37.956) -> (-87.4638, -37.956)
  spline S479 degree 3 poles (-87.4638, -37.956) (-87.7387, -37.956) (-87.9637, -37.7311) (-87.9637, -37.456) knots 14 14 14 14 15 15 15 15
  line L479 (-87.9637, -37.456) -> (-87.9637, -24.4562)
  spline S480 degree 3 poles (-87.9637, -24.4562) (-87.9637, -24.1811) (-87.7387, -23.9562) (-87.4638, -23.9562) knots 16 16 16 16 17 17 17 17
  line L480 (-87.4638, -23.9562) -> (-53.0318, -23.9562)
  spline S481 degree 3 poles (-53.0318, -23.9562) (-52.7565, -23.9562) (-52.5315, -24.1811) (-52.5315, -24.4562) knots 18 18 18 18 19 19 19 19
  line L481 (-52.5315, -24.4562) -> (-52.5315, -37.456)
  spline S482 degree 3 poles (-100.1566, -56.506) (-100.1566, -56.7811) (-100.3815, -57.006) (-100.6568, -57.006) knots 0 0 0 0 1 1 1 1
  line L482 (-100.6568, -57.006) -> (-113.6569, -57.006)
  spline S483 degree 3 poles (-113.6569, -57.006) (-113.9318, -57.006) (-114.1568, -56.7811) (-114.1568, -56.506) knots 2 2 2 2 3 3 3 3
  line L483 (-114.1568, -56.506) -> (-114.1568, -43.5062)
  spline S484 degree 3 poles (-114.1568, -43.5062) (-114.1568, -43.2312) (-113.9318, -43.0062) (-113.6569, -43.0062) knots 4 4 4 4 5 5 5 5
  line L484 (-113.6569, -43.0062) -> (-100.6568, -43.0062)
  spline S485 degree 3 poles (-100.6568, -43.0062) (-100.3815, -43.0062) (-100.1566, -43.2312) (-100.1566, -43.5062) knots 6 6 6 6 7 7 7 7
  line L485 (-100.1566, -43.5062) -> (-100.1566, -56.506)
  spline S486 degree 3 poles (137.9686, -37.456) (137.9686, -37.7311) (137.7436, -37.956) (137.4684, -37.956) knots 0 0 0 0 1 1 1 1
  line L486 (137.4684, -37.956) -> (124.4686, -37.956)
  spline S487 degree 3 poles (124.4686, -37.956) (124.1937, -37.956) (123.9687, -37.7311) (123.9687, -37.456) knots 2 2 2 2 3 3 3 3
  line L487 (123.9687, -37.456) -> (123.9687, -24.4562)
  spline S488 degree 3 poles (123.9687, -24.4562) (123.9687, -24.1811) (124.1937, -23.9562) (124.4686, -23.9562) knots 4 4 4 4 5 5 5 5
  line L488 (124.4686, -23.9562) -> (137.4684, -23.9562)
  spline S489 degree 3 poles (137.4684, -23.9562) (137.7436, -23.9562) (137.9686, -24.1811) (137.9686, -24.4562) knots 6 6 6 6 7 7 7 7
  line L489 (137.9686, -24.4562) -> (137.9686, -37.456)
  spline S490 degree 3 poles (-119.2066, 43.5059) (-119.2066, 43.2308) (-119.4315, 43.0058) (-119.7068, 43.0058) knots 0 0 0 0 1 1 1 1
  line L490 (-119.7068, 43.0058) -> (-132.7069, 43.0058)
  spline S491 degree 3 poles (-132.7069, 43.0058) (-132.9818, 43.0058) (-133.2068, 43.2308) (-133.2068, 43.5059) knots 2 2 2 2 3 3 3 3
  line L491 (-133.2068, 43.5059) -> (-133.2068, 56.506)
  spline S492 degree 3 poles (-133.2068, 56.506) (-133.2068, 56.7811) (-132.9818, 57.006) (-132.7069, 57.006) knots 4 4 4 4 5 5 5 5
  line L492 (-132.7069, 57.006) -> (-119.7068, 57.006)
  spline S493 degree 3 poles (-119.7068, 57.006) (-119.4315, 57.006) (-119.2066, 56.7811) (-119.2066, 56.506) knots 6 6 6 6 7 7 7 7
  line L493 (-119.2066, 56.506) -> (-119.2066, 43.5059)
  spline S494 degree 3 poles (-100.1566, 0.6441) (-100.1566, 0.369) (-100.3815, 0.144) (-100.6568, 0.144) knots 0 0 0 0 1 1 1 1
  line L494 (-100.6568, 0.144) -> (-113.6569, 0.144)
  spline S495 degree 3 poles (-113.6569, 0.144) (-113.9318, 0.144) (-114.1568, 0.369) (-114.1568, 0.6441) knots 2 2 2 2 3 3 3 3
  line L495 (-114.1568, 0.6441) -> (-114.1568, 13.6438)
  spline S496 degree 3 poles (-114.1568, 13.6438) (-114.1568, 13.9189) (-113.9318, 14.1438) (-113.6569, 14.1438) knots 4 4 4 4 5 5 5 5
  line L496 (-113.6569, 14.1438) -> (-100.6568, 14.1438)
  spline S497 degree 3 poles (-100.6568, 14.1438) (-100.3815, 14.1438) (-100.1566, 13.9189) (-100.1566, 13.6438) knots 6 6 6 6 7 7 7 7
  line L497 (-100.1566, 13.6438) -> (-100.1566, 0.6441)
extrude "押し出し1'" add sketch "スケッチ1 (2)" along normal blind 2 separate body makes body 2 in component "CasePlateExtended"
sketch "スケッチ1 (3)" plane through (0, 0, 0) normal (0, 0, 1) x (1, 0, 0) in component "CaseTop"
  line L0 (193.3816, 60.0319) -> (193.3816, 39.9807)
  line L1 (-174.3318, 60.0319) -> (-97.1316, 60.0319)
  spline S0 degree 3 poles (-183.3569, 57.5059) (-179.2147, 57.5059) (-175.8569, 54.148) (-175.8569, 50.0056) (-175.8569, 45.8639) (-179.2147, 42.506) (-183.3569, 42.506) (-187.4991, 42.506) (-190.8569, 45.8639) (-190.8569, 50.0056) (-190.8569, 54.148) (-187.4991, 57.5059) (-183.3569, 57.5059) knots 0 0 0 0 1 1 1 2 2 2 3 3 3 4 4 4 4
  line L2 (-201.3816, 68.0317) -> (-201.3816, -68.0317)
  line L3 (-193.3816, 40.9808) -> (-174.3318, 40.9808)
  line L4 (-201.3816, -68.0317) -> (201.3818, -68.0317)
  line L5 (-97.1318, 17.169) -> (-97.1316, -60.0322)
  line L6 (193.3816, -60.0322) -> (-93.3697, -60.0322)
  line L7 (-93.3697, 36.2187) -> (193.3816, 36.2187)
  line L8 (193.3816, 36.2187) -> (193.3816, -60.0322)
  line L9 (193.3816, 39.9807) -> (-93.3697, 39.9807)
  line L10 (-174.3318, 40.9808) -> (-174.3318, 60.0319)
  line L11 (-97.1318, 20.9307) -> (-193.3816, 20.9307)
  line L12 (-193.3816, 17.169) -> (-97.1318, 17.169)
  line L13 (-193.3816, 20.9307) -> (-193.3816, 40.9808)
  line L14 (-93.3697, -60.0322) -> (-93.3697, 36.2187)
  line L15 (-97.1316, 60.0319) -> (-97.1318, 20.9307)
  line L16 (201.3818, -68.0317) -> (201.3818, 68.0317)
  line L17 (-97.1316, -60.0322) -> (-193.3816, -60.0322)
  line L18 (-93.3697, 39.9807) -> (-93.3697, 60.0319)
  line L19 (-193.3816, -60.0322) -> (-193.3816, 17.169)
  line L20 (-93.3697, 60.0319) -> (193.3816, 60.0319)
  line L21 (201.3818, 68.0317) -> (-201.3816, 68.0317)
extrude "押し出し1''" add sketch "スケッチ1 (3)" along normal blind 8 separate body makes body 3 in component "CaseTop"
move_body "移動1" bodies 3 to x (1, 0, 0) y (0, 1, 0) z (0, 0, 1) at (0, 0, 2) in component "CaseTop"
sketch "スケッチ1 (4)" plane through (0, 0, 0) normal (0, 0, 1) x (1, 0, 0) in component "CaseBottom"
  line L0 (201.3816, -68.0319) -> (201.3816, 68.0319)
  line L1 (-201.3816, -68.0319) -> (201.3816, -68.0319)
  line L2 (-201.3816, 68.0319) -> (-201.3816, -68.0319)
  line L3 (201.3816, 68.0319) -> (-201.3816, 68.0319)
extrude "押し出し1'''" add sketch "スケッチ1 (4)" along normal blind 12 separate body makes body 4 in component "CaseBottom"
move_body "移動1'" bodies 4 to x (1, 0, 0) y (0, 1, 0) z (0, 0, 1) at (0, 0, -12) in component "CaseBottom"
sketch "スケッチ2" plane through (0, 0, 0) normal (0, 0, 1) x (1, 0, 0) in component "CaseBottom"
  line L0 (-193.8817, -60.5321) -> (193.8817, -60.5321)
  line L1 (193.8817, 60.5321) -> (-193.8817, 60.5321)
  line L2 (193.8817, -60.5321) -> (193.8817, 60.5321)
  line L3 (-193.8817, 60.5321) -> (-193.8817, -60.5321)
extrude "押し出し2" add sketch "スケッチ2" along normal blind 10 separate body makes body 5 in component "CaseBottom"
move_body "移動2" bodies 5 to x (1, 0, 0) y (0, 1, 0) z (0, 0, 1) at (0, 0, -9) in component "CaseBottom"
sketch "スケッチ3" plane through (0, 0, 0) normal (0, 0, 1) x (1, 0, 0) in component "CaseBottom"
  line L0 (4.9053, 14.0689) -> (-19.1949, 14.0689)
  line L1 (-19.1949, 14.0689) -> (-19.1949, 74.0689)
  line L2 (-19.1949, 74.0689) -> (4.9053, 74.0689)
  line L3 (4.9053, 74.0689) -> (4.9053, 14.0689)
extrude "押し出し3" add sketch "スケッチ3" along normal blind 15 separate body makes body 6 in component "CaseBottom"
move_body "移動3" bodies 6 to x (1, 0, 0) y (0, 1, 0) z (0, 0, 1) at (0, 0, -13) in component "CaseBottom"
combine "結合1" operation cut target body 4 tool bodies 5 6 in component "CaseBottom"
sketch "スケッチ1 (5)" plane through (0, 0, 0) normal (0, 0, 1) x (1, 0, 0) in component "CaseBottomPlate"
  spline S0 degree 3 poles (12.9052, 7.069) (12.9052, 6.519) (12.4552, 6.0691) (11.9051, 6.0691) knots 0 0 0 0 1 1 1 1
  line L0 (11.9051, 6.0691) -> (-26.1948, 6.0691)
  spline S1 degree 3 poles (-26.1948, 6.0691) (-26.7448, 6.0691) (-27.1947, 6.519) (-27.1947, 7.069) knots 2 2 2 2 3 3 3 3
  line L1 (-27.1947, 7.069) -> (-27.1947, 67.0321)
  spline S2 degree 3 poles (-27.1947, 67.0321) (-27.1947, 67.5821) (-26.7448, 68.0321) (-26.1948, 68.0321) knots 4 4 4 4 5 5 5 5
  line L2 (-26.1948, 68.0321) -> (11.9051, 68.0321)
  spline S3 degree 3 poles (11.9051, 68.0321) (12.4552, 68.0321) (12.9052, 67.5821) (12.9052, 67.0321) knots 6 6 6 6 7 7 7 7
  line L3 (12.9052, 67.0321) -> (12.9052, 7.069)
extrude "押し出し1''''" add sketch "スケッチ1 (5)" along normal blind 2 separate body makes body 7 in component "CaseBottomPlate"
move_body "移動1''" bodies 7 to x (1, 0, 0) y (0, 1, 0) z (0, 0, 1) at (0, 0, -16) in component "CaseBottomPlate"